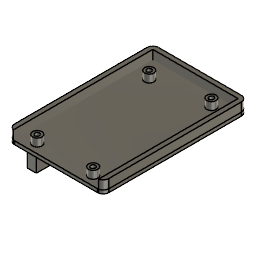
arduinoMount4040 (Autodesk Fusion 360 design; units mm, degrees)
part number: 2026-01-29-15-29-34-594
Autodesk Fusion 360 part; units mm, degrees
sketch "Sketch5" plane through (0, 0, 0) normal (0, 0, 1) x (1, 0, 0)
  line L0 (-41, -62.5) -> (41, -62.5)
  line L1 (41, -62.5) -> (41, 62.5)
  line L2 (41, 62.5) -> (-41, 62.5)
  line L3 (-41, 62.5) -> (-41, -62.5)
  line L4 (-41, -62.5) -> (41, 62.5) construction
  line L5 (41, -62.5) -> (-41, 62.5) construction
  line L6 (-37, 62.5) -> (-37, -62.5)
  line L7 (0, 62.5) -> (0, -62.5) construction
  line L8 (37, 62.5) -> (37, -62.5)
  line L9 (-10, -62.5) -> (10, -62.5) construction
  line L10 (-17.05, -62.5) -> (-24.95, -62.5)
  line L11 (-24.95, -62.5) -> (-24.95, 62.5)
  line L12 (-17.05, 62.5) -> (-17.05, -62.5)
  line L13 (-41, -58.5) -> (41, -58.5)
  line L14 (-27, -62.5) -> (-13, -62.5)
  circle A0 centre (-24.25, -54.5) radius 4
  circle A1 centre (-24.25, -54.5) radius 2
  circle A2 centre (-23.75, 42.2) radius 4
  circle A3 centre (-23.75, 42.2) radius 2
  circle A4 centre (24.25, -54.5) radius 4
  circle A5 centre (24.25, -54.5) radius 2
  circle A6 centre (23.95, 48.5) radius 4
  circle A7 centre (23.95, 48.5) radius 2
  line L15 (-23.75, 42.2) -> (-23.75, 42.0006) construction
  line L16 (21.9749, 48.8148) -> (24.5692, 48.8148) construction
  line L17 (24.25, -54.5) -> (24.25, 62.5) construction
  line L18 (-24.25, -54.5) -> (-24.25, -56.7551) construction
  line L19 (23.95, 48.5) -> (23.95, 47.5108) construction
  line L20 (-21, -62.5) -> (-21, 62.5) construction
  line L21 (-41, 58.5) -> (41, 58.5)
  line L22 (-25.25, -56.2321) -> (-24.25, -56.8094)
  line L23 (-25.25, -56.2321) -> (-22.671, -56.2321) construction
  line L24 (-23.25, -56.2321) -> (-24.25, -56.8094)
  line L25 (24.25, -54.5) -> (24.25, -55.6656) construction
  line L26 (23.25, -56.2321) -> (24.25, -56.8094)
  line L27 (23.25, -56.2321) -> (24.8251, -56.2321) construction
  line L28 (25.25, -56.2321) -> (24.25, -56.8094)
  line L29 (22.95, 46.7679) -> (23.95, 46.1906)
  line L30 (22.95, 46.7679) -> (25.4647, 46.7679) construction
  line L31 (24.95, 46.7679) -> (23.95, 46.1906)
  line L32 (-24.75, 40.4679) -> (-23.75, 39.8906)
  line L33 (-24.75, 40.4679) -> (-23.1842, 40.4679) construction
  line L34 (-22.75, 40.4679) -> (-23.75, 39.8906)
  dimension "d29" = 125
  dimension "d30" = 4
  dimension "d55" = 7.9
  dimension "d93" = 74
  dimension "d94" = 4
  dimension "d101" = 4
  dimension "d103" = 14
  dimension "d116" = 8
  dimension "d117" = 4
  dimension "d118" = 8
  dimension "d119" = 4
  dimension "d120" = 8
  dimension "d121" = 4
  dimension "d122" = 8
  dimension "d123" = 4
  dimension "d124" = 48.5
  dimension "d127" = 24.25
  dimension "d128" = 4
  dimension "d129" = 96.7
  dimension "d132" = 103
  dimension "d135" = 0.3
  dimension "d136" = 0.5
  dimension "d146" = 20
  dimension "d147" = 3.95
  dimension "d151" = 4
  dimension "d156" = 30
  dimension "d157" = 30
  dimension "d158" = 30
  dimension "d159" = 30
  dimension "d160" = 121
  dimension "d161" = 82
  constraint horizontal L0
  constraint perpendicular L0 L1
  constraint parallel L0 L2
  constraint parallel L1 L3
  constraint coincident L4 origin
  constraint coincident L5 origin
  constraint coincident L2 L6.start
  constraint coincident L0 L6.end
  constraint perpendicular L0 L6
  constraint midpoint L2 L7.start
  constraint midpoint L0 L7.end
  constraint symmetric L6.start L7 L8.start
  constraint symmetric L6.end L7 L8.end
  constraint horizontal L9
  constraint coincident L0 L9.start
  constraint horizontal L10
  constraint vertical L11
  constraint vertical L12
  constraint coincident L0 L10.start
  constraint coincident L3 L13.start
  constraint coincident L1 L13.end
  constraint perpendicular L1 L13
  constraint horizontal L14
  constraint coincident L0 L14.start
  constraint concentric A0 A1
  constraint concentric A2 A3
  constraint concentric A4 A5
  constraint concentric A6 A7
  constraint horizontal A0.centre A4.centre
  constraint vertical L15
  constraint coincident A2.centre A3.centre
  constraint horizontal L16
  constraint coincident A7 L16.start
  constraint vertical L17
  constraint coincident A4.centre A5.centre
  constraint vertical L18
  constraint coincident A0.centre A1.centre
  constraint coincident L2 L17.end
  constraint vertical L19
  constraint coincident A6.centre A7.centre
  constraint coincident L0 L20.start
  constraint coincident L2 L20.end
  constraint perpendicular L2 L20
  constraint coincident L2 L11.end
  constraint coincident L2 L12.start
  constraint coincident L3 L21.start
  constraint coincident L1 L21.end
  constraint perpendicular L1 L21
  constraint horizontal L23
  constraint coincident A1 L22.start
  constraint tangent A1 L22
  constraint coincident L18 L22.end
  constraint symmetric L18 L22.start L24.start
  constraint symmetric L18 L22.end L24.end
  constraint parallel L17 L25
  constraint horizontal L27
  constraint coincident A5 L26.start
  constraint tangent A5 L26
  constraint coincident L25 L26.end
  constraint symmetric L25 L26.start L28.start
  constraint symmetric L25 L26.end L28.end
  constraint horizontal L30
  constraint coincident A7 L29.start
  constraint tangent A7 L29
  constraint coincident L19 L29.end
  constraint symmetric L19 L29.start L31.start
  constraint symmetric L19 L29.end L31.end
  constraint horizontal L33
  constraint coincident A3 L32.start
  constraint tangent A3 L32
  constraint coincident L15 L32.end
  constraint symmetric L15 L32.start L34.start
  constraint symmetric L15 L32.end L34.end
  measures "d29" distance of L0.end L1.end
  measures "d30" distance of L3 L6
  measures "d55" distance of L10.start L10.end
  measures "d93" distance of L6 L8
  measures "d94" distance of L1 L8
  measures "d101" distance of L0 L13
  measures "d103" distance of L14.start L14.end
  measures "d116" diameter of A0
  measures "d117" diameter of A1
  measures "d118" diameter of A2
  measures "d119" diameter of A3
  measures "d120" diameter of A4
  measures "d121" diameter of A5
  measures "d122" diameter of A6
  measures "d123" diameter of A7
  measures "d124" horizontal distance of A0.centre A4.centre
  measures "d127" distance of L7 A4.centre
  measures "d128" distance of L13 A4.centre
  measures "d129" vertical distance of A0.centre A2.centre
  measures "d132" vertical distance of A4.centre A6.centre
  measures "d135" horizontal distance of A4.centre A6.centre
  measures "d136" horizontal distance of A0.centre A2.centre
  measures "d146" distance of L3 L20
  measures "d147" distance of L11 L20
  measures "d151" distance of L2 L21
  measures "d156" angle of L22 L23
  measures "d157" angle of L26 L27
  measures "d158" angle of L29 L30
  measures "d159" angle of L32 L33
  measures "d160" distance of L0 L21
  measures "d161" distance of L1 L3
sketch "Sketch6" plane through (0, 0, 0) normal (0, 1, 0) x (1, 0, 0)
  line L0 (0, -56.6756) -> (0, 40) construction
  line L1 (-20, 40) -> (-20, 0) construction
  line L2 (20, 40) -> (20, 0) construction
  line L3 (20, 40) -> (20, 0) construction
  point P0 (0, -10.7)
  point P1 (0, -9.7)
  point P2 (0, -56.6756)
  point P3 (0, 40)
  point P4 (-20, 16)
  point P5 (20, 16)
  point P6 (-20, 12)
  point P7 (-20, 5)
  point P8 (20, 16)
  point P9 (20, 5)
  point P10 (-20, 24)
  point P11 (20, 24)
  point P12 (-24.75, 0)
  point P13 (-37, 0)
  point P14 (20, 24)
  point P15 (20, 12)
  point P16 (37, 0)
  point P17 (20, 16)
  point P18 (24.75, 0)
  point P19 (20, 5)
  point P20 (0, -3)
  dimension "d36" = 40
  dimension "d45" = 20
  dimension "d46" = 20
  dimension "d48" = 40
  dimension "d49" = 12
  dimension "d50" = 5
  dimension "d51" = 16
  dimension "d52" = 8
  dimension "d53" = 16
  dimension "d54" = 12.25
  dimension "d100" = 1
  dimension "d164" = 3
  dimension "d165" = 6.7
  constraint vertical P0 P1
  constraint vertical P1 origin
  constraint coincident P2 L0.start
  constraint coincident P3 L0.end
  constraint vertical L0
  constraint horizontal P4 P17
  constraint horizontal P3 L1.start
  constraint vertical P4 L1.start
  constraint coincident L1 P6
  constraint coincident L1 P7
  constraint symmetric P4 L0 P17
  constraint symmetric L0 L1.start L2.start
  constraint symmetric L0 L1.end L2.end
  constraint symmetric L0 P7 P19
  constraint coincident L1 P10
  constraint symmetric L0 P10 P14
  constraint symmetric L0 P6 P15
  constraint symmetric L0 P12 P18
  constraint symmetric L0 P13 P16
  constraint coincident L0 P20
  measures "d36" distance of P3 origin
  measures "d45" distance of P4 L0
  measures "d46" distance of P17 L0
  measures "d48" distance of L1.start L1.end
  measures "d49" distance of L1.end P6
  measures "d50" distance of L1.end P7
  measures "d51" distance of P4 L1.end
  measures "d52" distance of P4 P10
  measures "d53" distance of L1.start P10
  measures "d54" distance of P12 P13
  measures "d100" distance of P0 P1
  measures "d164" distance of origin P20
  measures "d165" distance of P1 P20
extrude "Extrude10" add sketch "Sketch5" along normal up to surface (3 mm away) contours L0 L3 L6 L13 | L0 L6 L11 L13 L14 | L3 L6 L13 L21 | L6 L11 L13 A0 A2 L21 | L2 L3 L6 L21 | L0 L10 L11 L12 L13 L14 | L2 L6 L11 L21 | L11 L13 A0 | L0 L8 L12 L13 L14 | L11 L12 L13 A0 A2 L21 | L2 L11 L12 L21 | L11 A0 A1 L22 | L11 A0 A1 L22 L24 | A4 | L8 L12 L13 L21 | L11 A2 A3 L32 L34 | L11 A2 A3 | L2 L8 L12 L21 | L11 A1 L22 | L11 A1 L22 L24 | L0 L1 L8 L13 | L11 A3 | L11 A3 | L1 L8 L13 L21 | L1 L2 L8 L21 | L11 A1 | L11 A1 | A3 L32 L34 | A5 | A5 L26 L28 | A6 | A7 | A7 L29 L31 makes body 1
extrude "Extrude21" add sketch "Sketch5" along normal up to surface (6.7 mm away) from surface at 3 separate body contours L11 A0 A1 L22 | L11 A0 A1 L22 L24 | A4 | L11 A2 A3 L32 L34 | L11 A2 A3 | A6 makes body 2 at (28.2301, -54.1017, 7.4667) makes body 3 at (-19.7699, 41.8017, 5.2333) makes body 4 at (-20.2699, -54.1017, 7.4667) makes body 5 at (27.9301, 48.1017, 7.4667)
extrude "Extrude14" add sketch "Sketch5" against normal up to surface (12 mm away) separate body contours L0 L10 L11 L12 L13 L14 | L11 L13 A0 | L11 L12 L13 A0 A2 L21 | L2 L11 L12 L21 | L11 A0 A1 L22 L24 | L11 A2 A3 L32 L34 | L11 A1 L22 L24 | L11 A3 | L11 A1 | A3 L32 L34 picked at (-23.9781, 41.5828) picked at (-24.0816, -53.9065) makes body 6
sketch "Sketch8" plane through (-17.05, 0, 0) normal (1, 0, 0) x (0, 1, 0)
  line L0 (-62.5, -5) -> (62.5, -5)
  line L1 (62.5, -5) -> (-62.5, -5)
  line L2 (-62.5, -12) -> (62.5, -12)
  line L3 (62.5, -12) -> (62.5, 0)
  line L4 (62.5, 0) -> (-62.5, 0)
  line L5 (-62.5, 0) -> (-62.5, -12)
  dimension "d149" = 5
  constraint coincident L0.start L5
  constraint coincident L0.end L3
  measures "d149" distance of L1 L4
extrude "Extrude15" [suppressed]
fillet "Fillet1" [suppressed]
sketch "Sketch9" plane through (-24.95, 0, 0) normal (-1, 0, 0) x (0, -1, 0)
  line L0 (-62.5, -5) -> (62.5, -5)
  line L1 (-62.5, -12) -> (62.5, -12)
  line L2 (62.5, -12) -> (62.5, 0)
  line L3 (62.5, 0) -> (-62.5, 0)
  line L4 (-62.5, 0) -> (-62.5, -12)
  dimension "d150" = 5
  constraint coincident L0.end L2
  constraint coincident L0.start L4
  measures "d150" distance of L0 L3
extrude "Extrude16" [suppressed]
fillet "Fillet2" [suppressed]
extrude "Extrude20" add sketch "Sketch5" along normal up to surface (10.7 mm away) separate body contours L0 L3 L6 L13 | L3 L6 L13 L21 | L2 L3 L6 L21 | L2 L6 L11 L21 | L2 L11 L12 L21 | L2 L8 L12 L21 | L0 L1 L8 L13 | L1 L8 L13 L21 | L1 L2 L8 L21 makes body 7
fillet "Fillet7" radius 5 8 edges at (41, 62.5, 1.5) (41, -62.5, 1.5) (-41, -62.5, 1.5) (-41, 62.5, 1.5) (41, -62.5, 5.35) (41, 62.5, 5.35) (-41, -62.5, 5.35) (-41, 62.5, 5.35) on bodies 1 7
equation "d46 = d45"
equation "d47 = 8 mm"
equation "d51 = d48 / 2 - d47 / 2"
equation "d101 = d30"
equation "d116 = d118"
equation "d118 = d117 + 4 mm"
equation "d120 = d118"
equation "d122 = d118"
equation "d127 = d124 / 2"
equation "d147 = d55 / 2"
equation "d149 = d50"
equation "d150 = d50"
equation "d151 = d101"
